Autodesk Fusion 360 part; units mm, degrees
(part 2 of 2)
  spline S93 degree 3 poles (-0.4829, 17.1605) (-0.5355, 17.2267) (-0.6438, 17.3632) (-0.6565, 17.5373) (-0.663, 17.6271) knots 0 0 0 0 0.024747 0.051056 0.051056 0.051056 0.051056
  spline S94 degree 3 poles (-0.663, 17.6271) (-0.6569, 17.7139) (-0.645, 17.8842) (-0.5509, 18.0265) (-0.5048, 18.0964) knots 0 0 0 0 0.025614 0.050281 0.050281 0.050281 0.050281
  spline S95 degree 3 poles (-0.5048, 18.0964) (-0.4337, 18.1672) (-0.2885, 18.3119) (-0.0839, 18.33) (0.0205, 18.3392) knots 0 0 0 0 0.029141 0.059529 0.059529 0.059529 0.059529
  line L42 (4.4066, 19.7731) -> (4.2483, 19.7731)
  line L43 (4.2483, 19.7731) -> (4.2483, 21.7813)
  line L44 (4.2483, 21.7813) -> (4.4939, 21.7813)
  line L45 (4.4939, 21.7813) -> (4.4939, 20.2164)
  spline S96 degree 3 poles (4.4939, 20.2164) (4.5274, 20.2456) (4.5999, 20.3087) (4.6822, 20.3587) (4.7265, 20.3856) knots 0 0 0 0 0.013289 0.028808 0.028808 0.028808 0.028808
  spline S97 degree 3 poles (4.7265, 20.3856) (4.7715, 20.4114) (4.855, 20.4592) (4.944, 20.4957) (4.985, 20.5125) knots 0 0 0 0 0.015536 0.028826 0.028826 0.028826 0.028826
  line L46 (4.985, 20.5125) -> (4.985, 20.2751)
  spline S98 degree 3 poles (4.985, 20.2751) (4.9192, 20.2417) (4.7906, 20.1765) (4.6792, 20.0851) (4.6249, 20.0405) knots 0 0 0 0 0.022076 0.0431 0.0431 0.0431 0.0431
  spline S99 degree 3 poles (4.6249, 20.0405) (4.5785, 19.9972) (4.4934, 19.918) (4.4337, 19.8184) (4.4066, 19.7731) knots 0 0 0 0 0.01891 0.03467 0.03467 0.03467 0.03467
  spline S100 degree 3 poles (-4.5976, 21.8167) (-4.5145, 21.8111) (-4.3537, 21.8001) (-4.2234, 21.7056) (-4.1603, 21.6598) knots 0 0 0 0 0.024413 0.047298 0.047298 0.047298 0.047298
  spline S101 degree 3 poles (-4.1603, 21.6598) (-4.1085, 21.6029) (-4.0028, 21.4869) (-3.9757, 21.3321) (-3.9618, 21.2533) knots 0 0 0 0 0.022603 0.04608 0.04608 0.04608 0.04608
  line L47 (-3.9618, 21.2533) -> (-4.2074, 21.2205)
  spline S102 degree 3 poles (-4.2074, 21.2205) (-4.2215, 21.2828) (-4.2469, 21.3945) (-4.3193, 21.4825) (-4.3513, 21.5214) knots 0 0 0 0 0.018844 0.033755 0.033755 0.033755 0.033755
  spline S103 degree 3 poles (-4.3513, 21.5214) (-4.3875, 21.5482) (-4.461, 21.6029) (-4.5524, 21.6099) (-4.5989, 21.6134) knots 0 0 0 0 0.01322 0.026904 0.026904 0.026904 0.026904
  spline S104 degree 3 poles (-4.5989, 21.6134) (-4.6543, 21.6086) (-4.7643, 21.5989) (-4.8493, 21.5284) (-4.8916, 21.4934) knots 0 0 0 0 0.016258 0.032307 0.032307 0.032307 0.032307
  spline S105 degree 3 poles (-4.8916, 21.4934) (-4.9264, 21.4506) (-4.9969, 21.3639) (-5.0062, 21.2524) (-5.0109, 21.196) knots 0 0 0 0 0.016147 0.032721 0.032721 0.032721 0.032721
  spline S106 degree 3 poles (-5.0109, 21.196) (-5.0068, 21.1425) (-4.9986, 21.038) (-4.9327, 20.9567) (-4.9004, 20.917) knots 0 0 0 0 0.015678 0.030648 0.030648 0.030648 0.030648
  spline S107 degree 3 poles (-4.9004, 20.917) (-4.8604, 20.885) (-4.7783, 20.8193) (-4.6732, 20.8113) (-4.6194, 20.8072) knots 0 0 0 0 0.015012 0.030805 0.030805 0.030805 0.030805
  spline S108 degree 3 poles (-4.6194, 20.8072) (-4.5933, 20.8087) (-4.5347, 20.8122) (-4.4777, 20.8265) (-4.4461, 20.8345) knots 0 0 0 0 0.00784 0.017573 0.017573 0.017573 0.017573
  line L48 (-4.4461, 20.8345) -> (-4.4734, 20.6189)
  spline S109 degree 3 poles (-4.4734, 20.6189) (-4.4808, 20.6197) (-4.494, 20.6211) (-4.5072, 20.6215) (-4.513, 20.6216) knots 0 0 0 0 0.002226 0.003967 0.003967 0.003967 0.003967
  spline S110 degree 3 poles (-4.513, 20.6216) (-4.5637, 20.6184) (-4.6639, 20.612) (-4.7519, 20.5637) (-4.7954, 20.5398) knots 0 0 0 0 0.015044 0.029725 0.029725 0.029725 0.029725
  spline S111 degree 3 poles (-4.7954, 20.5398) (-4.832, 20.5078) (-4.9081, 20.4411) (-4.9165, 20.34) (-4.9209, 20.2874) knots 0 0 0 0 0.014029 0.029194 0.029194 0.029194 0.029194
  spline S112 degree 3 poles (-4.9209, 20.2874) (-4.9173, 20.2446) (-4.9104, 20.1603) (-4.8561, 20.0955) (-4.8295, 20.0637) knots 0 0 0 0 0.012556 0.024703 0.024703 0.024703 0.024703
  spline S113 degree 3 poles (-4.8295, 20.0637) (-4.796, 20.0378) (-4.7266, 19.9842) (-4.6389, 19.9781) (-4.5935, 19.975) knots 0 0 0 0 0.012404 0.025721 0.025721 0.025721 0.025721
  spline S114 degree 3 poles (-4.5935, 19.975) (-4.5481, 19.9783) (-4.4596, 19.9849) (-4.3891, 20.0388) (-4.3547, 20.065) knots 0 0 0 0 0.013323 0.026012 0.026012 0.026012 0.026012
  spline S115 degree 3 poles (-4.3547, 20.065) (-4.3254, 20.1011) (-4.2612, 20.1801) (-4.2423, 20.2805) (-4.2319, 20.3351) knots 0 0 0 0 0.013719 0.030088 0.030088 0.030088 0.030088
  line L49 (-4.2319, 20.3351) -> (-3.9864, 20.2915)
  spline S116 degree 3 poles (-3.9864, 20.2915) (-4.0047, 20.2151) (-4.0397, 20.0694) (-4.1423, 19.9605) (-4.191, 19.9088) knots 0 0 0 0 0.023119 0.04407 0.04407 0.04407 0.04407
  spline S117 degree 3 poles (-4.191, 19.9088) (-4.2487, 19.8692) (-4.3683, 19.7873) (-4.5131, 19.7779) (-4.588, 19.7731) knots 0 0 0 0 0.020598 0.042654 0.042654 0.042654 0.042654
  spline S118 degree 3 poles (-4.588, 19.7731) (-4.6412, 19.7758) (-4.7459, 19.7812) (-4.8421, 19.8228) (-4.8895, 19.8433) knots 0 0 0 0 0.015821 0.03118 0.03118 0.03118 0.03118
  spline S119 degree 3 poles (-4.8895, 19.8433) (-4.9324, 19.8684) (-5.0164, 19.9174) (-5.0728, 19.9964) (-5.1003, 20.035) knots 0 0 0 0 0.014725 0.02878 0.02878 0.02878 0.02878
  spline S120 degree 3 poles (-5.1003, 20.035) (-5.1216, 20.0759) (-5.1637, 20.1568) (-5.1701, 20.2478) (-5.1733, 20.2928) knots 0 0 0 0 0.013662 0.027054 0.027054 0.027054 0.027054
  spline S121 degree 3 poles (-5.1733, 20.2928) (-5.1704, 20.335) (-5.1648, 20.4188) (-5.124, 20.4923) (-5.1037, 20.5289) knots 0 0 0 0 0.012502 0.024877 0.024877 0.024877 0.024877
  spline S122 degree 3 poles (-5.1037, 20.5289) (-5.0768, 20.5629) (-5.0205, 20.6342) (-4.9398, 20.6761) (-4.8977, 20.698) knots 0 0 0 0 0.012871 0.026927 0.026927 0.026927 0.026927
  spline S123 degree 3 poles (-4.8977, 20.698) (-4.953, 20.7146) (-5.0601, 20.7468) (-5.1364, 20.8284) (-5.1733, 20.8679) knots 0 0 0 0 0.016967 0.032892 0.032892 0.032892 0.032892
  spline S124 degree 3 poles (-5.1733, 20.8679) (-5.2019, 20.915) (-5.2621, 21.0139) (-5.2683, 21.1298) (-5.2715, 21.1905) knots 0 0 0 0 0.016275 0.034197 0.034197 0.034197 0.034197
  spline S125 degree 3 poles (-5.2715, 21.1905) (-5.2635, 21.2746) (-5.2474, 21.443) (-5.1362, 21.5707) (-5.0805, 21.6346) knots 0 0 0 0 0.024665 0.049435 0.049435 0.049435 0.049435
  spline S126 degree 3 poles (-5.0805, 21.6346) (-5.0113, 21.6877) (-4.869, 21.797) (-4.6897, 21.81) (-4.5976, 21.8167) knots 0 0 0 0 0.025577 0.052634 0.052634 0.052634 0.052634
  spline S127 degree 3 poles (0, 25.2779) (0.0905, 25.2701) (0.267, 25.2551) (0.3929, 25.131) (0.4543, 25.0705) knots 0 0 0 0 0.026334 0.051363 0.051363 0.051363 0.051363
  spline S128 degree 3 poles (0.4543, 25.0705) (0.5117, 24.9633) (0.6467, 24.7108) (0.6501, 24.423) (0.6521, 24.2574) knots 0 0 0 0 0.036009 0.08476 0.08476 0.08476 0.08476
  spline S129 degree 3 poles (0.6521, 24.2574) (0.6507, 24.1501) (0.6481, 23.9568) (0.6003, 23.7697) (0.5791, 23.6865) knots 0 0 0 0 0.032061 0.057736 0.057736 0.057736 0.057736
  spline S130 degree 3 poles (0.5791, 23.6865) (0.5533, 23.6197) (0.5043, 23.4931) (0.4078, 23.3979) (0.3622, 23.3529) knots 0 0 0 0 0.021191 0.040192 0.040192 0.040192 0.040192
  spline S131 degree 3 poles (0.3622, 23.3529) (0.3097, 23.3187) (0.1997, 23.2471) (0.0685, 23.2395) (0, 23.2356) knots 0 0 0 0 0.018481 0.038665 0.038665 0.038665 0.038665
  spline S132 degree 3 poles (0, 23.2356) (-0.0511, 23.2378) (-0.1493, 23.2421) (-0.2393, 23.2815) (-0.2824, 23.3004) knots 0 0 0 0 0.015196 0.029197 0.029197 0.029197 0.029197
  spline S133 degree 3 poles (-0.2824, 23.3004) (-0.3213, 23.3246) (-0.4002, 23.3739) (-0.4551, 23.4491) (-0.4829, 23.4873) knots 0 0 0 0 0.013619 0.027641 0.027641 0.027641 0.027641
  spline S134 degree 3 poles (-0.4829, 23.4873) (-0.5083, 23.5316) (-0.5619, 23.6256) (-0.5915, 23.7297) (-0.6071, 23.7847) knots 0 0 0 0 0.01527 0.032333 0.032333 0.032333 0.032333
  spline S135 degree 3 poles (-0.6071, 23.7847) (-0.6202, 23.8531) (-0.65, 24.0091) (-0.6514, 24.1681) (-0.6521, 24.2574) knots 0 0 0 0 0.020858 0.04757 0.04757 0.04757 0.04757
  spline S136 degree 3 poles (-0.6521, 24.2574) (-0.6507, 24.364) (-0.648, 24.5564) (-0.6008, 24.7426) (-0.5798, 24.8256) knots 0 0 0 0 0.031856 0.057454 0.057454 0.057454 0.057454
  spline S137 degree 3 poles (-0.5798, 24.8256) (-0.5541, 24.8924) (-0.5054, 25.0192) (-0.4091, 25.1147) (-0.3636, 25.1598) knots 0 0 0 0 0.021185 0.040213 0.040213 0.040213 0.040213
  spline S138 degree 3 poles (-0.3636, 25.1598) (-0.3109, 25.1942) (-0.2006, 25.2663) (-0.0689, 25.2739) (0, 25.2779) knots 0 0 0 0 0.018535 0.038823 0.038823 0.038823 0.038823
  arc A0 (6.725, 12.125) -> (6.925, 12.325) centre (6.725, 12.325) ccw
  line L50 (6.925, 12.325) -> (6.925, 25.775)
  arc A1 (6.925, 25.775) -> (6.725, 25.975) centre (6.725, 25.775) ccw
  line L51 (6.725, 25.975) -> (-6.725, 25.975)
  arc A2 (-6.725, 25.975) -> (-6.925, 25.775) centre (-6.725, 25.775) ccw
  line L52 (-6.925, 25.775) -> (-6.925, 12.325)
  arc A3 (-6.925, 12.325) -> (-6.725, 12.125) centre (-6.725, 12.325) ccw
  line L53 (-6.725, 12.125) -> (6.725, 12.125)
  spline S139 degree 3 poles (0.0027, 23.4388) (0.0564, 23.4451) (0.165, 23.4576) (0.2367, 23.5403) (0.2729, 23.5821) knots 0 0 0 0 0.015627 0.031586 0.031586 0.031586 0.031586
  spline S140 degree 3 poles (0.2729, 23.5821) (0.3095, 23.6678) (0.4012, 23.8822) (0.4003, 24.1166) (0.3997, 24.2574) knots 0 0 0 0 0.027708 0.069337 0.069337 0.069337 0.069337
  spline S141 degree 3 poles (0.3997, 24.2574) (0.4011, 24.3964) (0.4034, 24.6233) (0.3177, 24.832) (0.2844, 24.9129) knots 0 0 0 0 0.041114 0.067132 0.067132 0.067132 0.067132
  spline S142 degree 3 poles (0.2844, 24.9129) (0.2453, 24.9604) (0.1706, 25.051) (0.055, 25.0679) (0, 25.0759) knots 0 0 0 0 0.017756 0.03385 0.03385 0.03385 0.03385
  spline S143 degree 3 poles (0, 25.0759) (-0.055, 25.0679) (-0.1708, 25.0508) (-0.2453, 24.9599) (-0.2844, 24.9122) knots 0 0 0 0 0.016099 0.03389 0.03389 0.03389 0.03389
  spline S144 degree 3 poles (-0.2844, 24.9122) (-0.3177, 24.8313) (-0.4033, 24.6228) (-0.4011, 24.3961) (-0.3997, 24.2574) knots 0 0 0 0 0.026034 0.067063 0.067063 0.067063 0.067063
  spline S145 degree 3 poles (-0.3997, 24.2574) (-0.4012, 24.1181) (-0.4035, 23.8909) (-0.3177, 23.682) (-0.2844, 23.6012) knots 0 0 0 0 0.041199 0.067201 0.067201 0.067201 0.067201
  spline S146 degree 3 poles (-0.2844, 23.6012) (-0.245, 23.5539) (-0.1694, 23.4632) (-0.053, 23.4467) (0.0027, 23.4388) knots 0 0 0 0 0.01777 0.034058 0.034058 0.034058 0.034058
  line L54 (4.4407, 16.713) -> (5.0669, 17.6148)
  line L55 (5.0669, 17.6148) -> (4.4407, 17.6148)
  line L56 (4.4407, 17.6148) -> (4.4407, 16.713)
  spline S147 degree 3 poles (-4.6371, 17.2383) (-4.5838, 17.2432) (-4.477, 17.2532) (-4.3955, 17.3228) (-4.3547, 17.3576) knots 0 0 0 0 0.015669 0.031337 0.031337 0.031337 0.031337
  spline S148 degree 3 poles (-4.3547, 17.3576) (-4.3209, 17.4018) (-4.2503, 17.494) (-4.2427, 17.6102) (-4.2388, 17.6707) knots 0 0 0 0 0.016309 0.034061 0.034061 0.034061 0.034061
  spline S149 degree 3 poles (-4.2388, 17.6707) (-4.241, 17.7126) (-4.2456, 17.7965) (-4.2769, 17.8745) (-4.2927, 17.9136) knots 0 0 0 0 0.012488 0.025026 0.025026 0.025026 0.025026
  spline S150 degree 3 poles (-4.2927, 17.9136) (-4.3119, 17.9496) (-4.3493, 18.0196) (-4.4127, 18.0672) (-4.4434, 18.0902) knots 0 0 0 0 0.012088 0.023476 0.023476 0.023476 0.023476
  spline S151 degree 3 poles (-4.4434, 18.0902) (-4.4757, 18.1079) (-4.5392, 18.1427) (-4.6113, 18.1482) (-4.6467, 18.1509) knots 0 0 0 0 0.01092 0.021432 0.021432 0.021432 0.021432
  spline S152 degree 3 poles (-4.6467, 18.1509) (-4.6971, 18.1453) (-4.8002, 18.1336) (-4.8756, 18.062) (-4.9141, 18.0254) knots 0 0 0 0 0.014798 0.030269 0.030269 0.030269 0.030269
  spline S153 degree 3 poles (-4.9141, 18.0254) (-4.9467, 17.9777) (-5.0166, 17.8752) (-5.0227, 17.7508) (-5.0259, 17.6844) knots 0 0 0 0 0.017015 0.03652 0.03652 0.03652 0.03652
  spline S154 degree 3 poles (-5.0259, 17.6844) (-5.0227, 17.6205) (-5.0166, 17.5007) (-4.9476, 17.4031) (-4.9154, 17.3576) knots 0 0 0 0 0.018742 0.035129 0.035129 0.035129 0.035129
  spline S155 degree 3 poles (-4.9154, 17.3576) (-4.876, 17.3228) (-4.7963, 17.2526) (-4.6905, 17.2431) (-4.6371, 17.2383) knots 0 0 0 0 0.015362 0.030997 0.030997 0.030997 0.030997
  spline S156 degree 3 poles (-4.6112, 13.9613) (-4.6653, 13.9566) (-4.7718, 13.9474) (-4.852, 13.8767) (-4.8916, 13.8419) knots 0 0 0 0 0.01582 0.031195 0.031195 0.031195 0.031195
  spline S157 degree 3 poles (-4.8916, 13.8419) (-4.9236, 13.796) (-4.9926, 13.697) (-4.9983, 13.576) (-5.0014, 13.5111) knots 0 0 0 0 0.01645 0.035493 0.035493 0.035493 0.035493
  spline S158 degree 3 poles (-5.0014, 13.5111) (-4.998, 13.4458) (-4.9917, 13.323) (-4.9216, 13.2225) (-4.8888, 13.1755) knots 0 0 0 0 0.019171 0.036033 0.036033 0.036033 0.036033
  spline S159 degree 3 poles (-4.8888, 13.1755) (-4.8499, 13.1393) (-4.7732, 13.068) (-4.6692, 13.0568) (-4.618, 13.0513) knots 0 0 0 0 0.015505 0.030512 0.030512 0.030512 0.030512
  spline S160 degree 3 poles (-4.618, 13.0513) (-4.5647, 13.0575) (-4.4549, 13.0702) (-4.3743, 13.1461) (-4.3329, 13.185) knots 0 0 0 0 0.015674 0.03225 0.03225 0.03225 0.03225
  spline S161 degree 3 poles (-4.3329, 13.185) (-4.2975, 13.2344) (-4.2234, 13.3378) (-4.2156, 13.465) (-4.2115, 13.5316) knots 0 0 0 0 0.017846 0.037388 0.037388 0.037388 0.037388
  spline S162 degree 3 poles (-4.2115, 13.5316) (-4.2155, 13.5914) (-4.2232, 13.7065) (-4.2932, 13.798) (-4.3268, 13.8419) knots 0 0 0 0 0.017547 0.033771 0.033771 0.033771 0.033771
  spline S163 degree 3 poles (-4.3268, 13.8419) (-4.3676, 13.8767) (-4.4497, 13.9468) (-4.5572, 13.9564) (-4.6112, 13.9613) knots 0 0 0 0 0.015682 0.031535 0.031535 0.031535 0.031535
  spline S164 degree 3 poles (0.0055, 13.8781) (0.0603, 13.8825) (0.168, 13.8911) (0.2516, 13.9593) (0.2926, 13.9927) knots 0 0 0 0 0.016099 0.03158 0.03158 0.03158 0.03158
  spline S165 degree 3 poles (0.2926, 13.9927) (0.3259, 14.0337) (0.3935, 14.1173) (0.4021, 14.2246) (0.4065, 14.2792) knots 0 0 0 0 0.015466 0.031479 0.031479 0.031479 0.031479
  spline S166 degree 3 poles (0.4065, 14.2792) (0.4044, 14.3141) (0.4, 14.3848) (0.3713, 14.4496) (0.3568, 14.4824) knots 0 0 0 0 0.010409 0.021077 0.021077 0.021077 0.021077
  spline S167 degree 3 poles (0.3568, 14.4824) (0.3381, 14.5134) (0.3005, 14.5755) (0.2394, 14.6148) (0.2087, 14.6346) knots 0 0 0 0 0.010689 0.021477 0.021477 0.021477 0.021477
  spline S168 degree 3 poles (0.2087, 14.6346) (0.1753, 14.6503) (0.1083, 14.6818) (0.0343, 14.6862) (-0.0027, 14.6884) knots 0 0 0 0 0.01097 0.022 0.022 0.022 0.022
  spline S169 degree 3 poles (-0.0027, 14.6884) (-0.0583, 14.6842) (-0.1669, 14.676) (-0.2519, 14.6082) (-0.2933, 14.5752) knots 0 0 0 0 0.016312 0.031835 0.031835 0.031835 0.031835
  spline S170 degree 3 poles (-0.2933, 14.5752) (-0.3267, 14.5343) (-0.3951, 14.4505) (-0.4036, 14.3426) (-0.4079, 14.2874) knots 0 0 0 0 0.015466 0.031649 0.031649 0.031649 0.031649
  spline S171 degree 3 poles (-0.4079, 14.2874) (-0.4034, 14.2312) (-0.3945, 14.121) (-0.3243, 14.0358) (-0.2899, 13.994) knots 0 0 0 0 0.016467 0.032302 0.032302 0.032302 0.032302
  spline S172 degree 3 poles (-0.2899, 13.994) (-0.2475, 13.9602) (-0.1611, 13.8912) (-0.0508, 13.8825) (0.0055, 13.8781) knots 0 0 0 0 0.015878 0.032386 0.032386 0.032386 0.032386
  spline S173 degree 3 poles (0.0014, 13.05) (0.0458, 13.0534) (0.1328, 13.06) (0.2012, 13.1138) (0.2347, 13.14) knots 0 0 0 0 0.013054 0.025513 0.025513 0.025513 0.025513
  spline S174 degree 3 poles (0.2347, 13.14) (0.2617, 13.1713) (0.3154, 13.2334) (0.3234, 13.3151) (0.3274, 13.3556) knots 0 0 0 0 0.012093 0.023986 0.023986 0.023986 0.023986
  spline S175 degree 3 poles (0.3274, 13.3556) (0.3241, 13.4002) (0.3175, 13.4872) (0.2627, 13.5547) (0.236, 13.5875) knots 0 0 0 0 0.013093 0.025466 0.025466 0.025466 0.025466
  spline S176 degree 3 poles (0.236, 13.5875) (0.2025, 13.6137) (0.1328, 13.6682) (0.0444, 13.6744) (-0.0014, 13.6775) knots 0 0 0 0 0.012488 0.025912 0.025912 0.025912 0.025912
  spline S177 degree 3 poles (-0.0014, 13.6775) (-0.046, 13.6743) (-0.1328, 13.668) (-0.2009, 13.6142) (-0.234, 13.5882) knots 0 0 0 0 0.013101 0.025433 0.025433 0.025433 0.025433
  spline S178 degree 3 poles (-0.234, 13.5882) (-0.2604, 13.5566) (-0.3136, 13.4932) (-0.321, 13.4107) (-0.3247, 13.3692) knots 0 0 0 0 0.012047 0.024215 0.024215 0.024215 0.024215
  spline S179 degree 3 poles (-0.3247, 13.3692) (-0.3209, 13.3261) (-0.3135, 13.2406) (-0.2585, 13.1747) (-0.2312, 13.1421) knots 0 0 0 0 0.012649 0.025094 0.025094 0.025094 0.025094
  spline S180 degree 3 poles (-0.2312, 13.1421) (-0.1978, 13.1152) (-0.1298, 13.0606) (-0.0428, 13.0536) (0.0014, 13.05) knots 0 0 0 0 0.012558 0.025536 0.025536 0.025536 0.025536
sketch "Sketch1 (3)" plane through (0, 0, -5) normal (0, 0, -1) x (1, 0, 0) in component "Case"
  arc A0 (63.55, -96.125) -> (66.55, -93.125) centre (63.55, -93.125) ccw
  line L0 (66.55, -93.125) -> (66.55, 33.075)
  arc A1 (66.55, 33.075) -> (63.55, 36.075) centre (63.55, 33.075) ccw
  line L1 (63.55, 36.075) -> (-25.45, 36.075)
  arc A2 (-25.45, 36.075) -> (-28.45, 33.075) centre (-25.45, 33.075) ccw
  line L2 (-28.45, 33.075) -> (-28.45, -93.125)
  arc A3 (-28.45, -93.125) -> (-25.45, -96.125) centre (-25.45, -93.125) ccw
  line L3 (-25.45, -96.125) -> (63.55, -96.125)
  circle A4 centre (-18.45, -83.625) radius 2
  circle A5 centre (-18.45, -52.625) radius 2
  circle A6 centre (56.55, -52.625) radius 2
  circle A7 centre (-23.45, 31.075) radius 2
  circle A8 centre (-23.45, -91.125) radius 2
  circle A9 centre (61.55, 31.075) radius 2
  circle A10 centre (56.55, -83.625) radius 2
  line L4 (-10.025, 9.025) -> (10.025, 9.025)
  line L5 (10.025, 9.025) -> (10.025, 29.075)
  line L6 (10.025, 29.075) -> (48.125, 29.075)
  line L7 (48.125, 29.075) -> (48.125, -48.125)
  line L8 (48.125, -48.125) -> (-10.025, -48.125)
  line L9 (-10.025, -48.125) -> (-10.025, 9.025)
  line L10 (-16.95, -55.625) -> (55.05, -55.625)
  line L11 (55.05, -55.625) -> (55.05, -80.625)
  line L12 (55.05, -80.625) -> (-16.95, -80.625)
  line L13 (-16.95, -80.625) -> (-16.95, -55.625)
  circle A11 centre (61.55, -91.125) radius 2
  line L14 (61.55, -91.125) -> (61.55, 31.075)
  line L15 (61.55, 31.075) -> (-23.45, 31.075)
  line L16 (-23.45, 31.075) -> (-23.45, -91.125)
  line L17 (-23.45, -91.125) -> (61.55, -91.125)
  circle A12 centre (61.55, -91.125) radius 2.3
  circle A13 centre (-23.45, -91.125) radius 2.3
  circle A14 centre (-23.45, 31.075) radius 2.3
  circle A15 centre (61.55, 31.075) radius 2.3
  circle A16 centre (61.55, -91.125) radius 5.0139
  circle A17 centre (56.55, -83.625) radius 4
  circle A18 centre (-23.45, -91.125) radius 5.0139
  circle A19 centre (-23.45, 31.075) radius 5.0139
  circle A20 centre (61.55, 31.075) radius 5.0139
  dimension "d103" = 4.6
  dimension "d104" = 8
  constraint concentric A11 A12
  constraint concentric A8 A13
  constraint concentric A7 A14
  constraint concentric A9 A15
  constraint equal A14 A15
  constraint equal A13 A14
  constraint equal A12 A13
  constraint concentric A11 A16
  constraint concentric A10 A17
  constraint tangent A16 A17
  constraint concentric A13 A18
  constraint concentric A14 A19
  constraint concentric A15 A20
  constraint equal A19 A20
  constraint equal A18 A19
  constraint equal A16 A18
  measures "d103" diameter of A12
  measures "d104" diameter of A17
extrude "Extrude1''" add sketch "Sketch1 (3)" along normal blind 6 separate body contours A0 L0 L3 A16 | L0 L3 L14 L17 A12 A16 | L3 L17 A16 A18 | L0 L14 A16 A20 | L2 L3 L16 L17 A13 A18 | L14 L17 A12 A16 | L0 L1 L14 L15 A15 A20 | L2 A3 L3 A18 | L16 L17 A13 A18 | L0 A1 L1 A20 | L14 L15 A15 A20 | L2 L16 A18 A19 | L1 L15 A19 A20 | L1 L2 L15 L16 A14 A19 | L15 L16 A14 A19 | L1 A2 L2 A19 makes body 3 in component "Case"
sketch "Sketch2 (2)" plane through (0, 0, -11) normal (0, 0, -1) x (1, 0, 0) in component "Case"
  circle A0 centre (-23.45, 31.075) radius 2.3
  circle A1 centre (61.55, -91.125) radius 2.3
  circle A2 centre (61.55, 31.075) radius 2.3
  circle A3 centre (-23.45, -91.125) radius 2.3
  line L0 (56.5361, -91.125) -> (-18.4361, -91.125)
  arc A4 (-18.4361, -91.125) -> (-23.45, -86.1111) centre (-23.45, -91.125) ccw
  line L1 (-23.45, -86.1111) -> (-23.45, 26.0611)
  arc A5 (-23.45, 26.0611) -> (-18.4361, 31.075) centre (-23.45, 31.075) ccw
  line L2 (-18.4361, 31.075) -> (56.5361, 31.075)
  arc A6 (56.5361, 31.075) -> (61.55, 26.0611) centre (61.55, 31.075) ccw
  line L3 (61.55, 26.0611) -> (61.55, -86.1111)
  arc A7 (61.55, -86.1111) -> (56.5361, -91.125) centre (61.55, -91.125) ccw
  line L4 (-25.45, -96.125) -> (63.55, -96.125)
  arc A8 (63.55, -96.125) -> (66.55, -93.125) centre (63.55, -93.125) ccw
  line L5 (66.55, -93.125) -> (66.55, 33.075)
  arc A9 (66.55, 33.075) -> (63.55, 36.075) centre (63.55, 33.075) ccw
  line L6 (63.55, 36.075) -> (-25.45, 36.075)
  arc A10 (-25.45, 36.075) -> (-28.45, 33.075) centre (-25.45, 33.075) ccw
  line L7 (-28.45, 33.075) -> (-28.45, -93.125)
  arc A11 (-28.45, -93.125) -> (-25.45, -96.125) centre (-25.45, -93.125) ccw
extrude "Extrude2''" add sketch "Sketch2 (2)" along normal blind 60 contours A0 | A1 | A2 | A3 | L4 A8 L5 A9 L6 A10 L7 A11 bodies 3 in component "Case"
sketch "Sketch3" plane through (0, 0, -71) normal (0, 0, -1) x (1, 0, 0) in component "Case"
  line L0 (61.55, 26.0611) -> (61.55, -86.1111)
  arc A0 (61.55, -86.1111) -> (56.5361, -91.125) centre (61.55, -91.125) ccw
  line L1 (56.5361, -91.125) -> (-18.4361, -91.125)
  arc A1 (-18.4361, -91.125) -> (-23.45, -86.1111) centre (-23.45, -91.125) ccw
  line L2 (-23.45, -86.1111) -> (-23.45, 26.0611)
  arc A2 (-23.45, 26.0611) -> (-18.4361, 31.075) centre (-23.45, 31.075) ccw
  line L3 (-18.4361, 31.075) -> (56.5361, 31.075)
  arc A3 (56.5361, 31.075) -> (61.55, 26.0611) centre (61.55, 31.075) ccw
  arc A4 (-28.45, -93.125) -> (-25.45, -96.125) centre (-25.45, -93.125) ccw
  line L4 (-25.45, -96.125) -> (63.55, -96.125)
  arc A5 (63.55, -96.125) -> (66.55, -93.125) centre (63.55, -93.125) ccw
  line L5 (66.55, -93.125) -> (66.55, 33.075)
  arc A6 (66.55, 33.075) -> (63.55, 36.075) centre (63.55, 33.075) ccw
  line L6 (63.55, 36.075) -> (-25.45, 36.075)
  arc A7 (-25.45, 36.075) -> (-28.45, 33.075) centre (-25.45, 33.075) ccw
  line L7 (-28.45, 33.075) -> (-28.45, -93.125)
extrude "Extrude3" add sketch "Sketch3" along normal blind 5 contours L0 A0 L1 A1 L2 A2 L3 A3 | A4 L4 A5 L5 A6 L6 A7 L7 bodies 3 in component "Case"
sketch "Sketch4 (2)" plane through (0, 0, -71) normal (0, 0, 1) x (-1, 0, 0) in component "Case"
  arc A0 (-56.5361, -91.125) -> (-61.55, -86.1111) centre (-61.55, -91.125) ccw
  line L0 (-56.5361, -91.125) -> (18.4361, -91.125)
  arc A1 (23.45, -86.1111) -> (18.4361, -91.125) centre (23.45, -91.125) ccw
  line L1 (23.45, -86.1111) -> (23.45, 26.0611)
  arc A2 (18.4361, 31.075) -> (23.45, 26.0611) centre (23.45, 31.075) ccw
  line L2 (18.4361, 31.075) -> (-56.5361, 31.075)
  arc A3 (-61.55, 26.0611) -> (-56.5361, 31.075) centre (-61.55, 31.075) ccw
  line L3 (-61.55, 26.0611) -> (-61.55, -86.1111)
  line L4 (8.65, -53.1111) -> (-61.35, -53.1111)
  line L5 (-61.35, -53.1111) -> (-61.35, -83.1111)
  line L6 (-61.35, -83.1111) -> (8.65, -83.1111)
  line L7 (8.65, -83.1111) -> (8.65, -53.1111)
  line L8 (8.65, -53.1111) -> (-61.35, -83.1111) construction
  line L9 (-61.35, -53.1111) -> (8.65, -83.1111) construction
  line L10 (-61.35, -74.1111) -> (-53.35, -74.1111)
  line L11 (-53.35, -74.1111) -> (-53.35, -65.1111)
  line L12 (-53.35, -65.1111) -> (-61.35, -65.1111)
  line L13 (-61.35, -83.1111) -> (-61.55, -83.1111) construction
  line L14 (-61.55, -83.1111) -> (-61.55, -86.1111) construction
  line L15 (-61.55, -86.1111) -> (-61.35, -86.1111) construction
  line L16 (-61.35, -86.1111) -> (-61.35, -83.1111) construction
  line L17 (6.555, -81.1061) -> (-59.255, -81.1061) construction
  line L18 (-59.255, -81.1061) -> (-59.255, -55.1161) construction
  line L19 (-59.255, -55.1161) -> (6.555, -55.1161) construction
  line L20 (6.555, -55.1161) -> (6.555, -81.1061) construction
  line L21 (6.555, -81.1061) -> (-59.255, -55.1161) construction
  line L22 (-59.255, -81.1061) -> (6.555, -55.1161) construction
  circle A4 centre (6.555, -81.1061) radius 1.15
  circle A5 centre (-59.255, -81.1061) radius 1.15
  circle A6 centre (-59.255, -55.1161) radius 1.15
  circle A7 centre (6.555, -55.1161) radius 1.15
  circle A8 centre (6.555, -81.1061) radius 3.65
  circle A9 centre (-59.255, -81.1061) radius 3.65
  circle A10 centre (-59.255, -55.1161) radius 3.65
  circle A11 centre (6.555, -55.1161) radius 3.65
  circle A12 centre (13.855, -6.055) radius 3.65
  line L23 (13.855, -6.055) -> (13.855, -32.045) construction
  circle A13 centre (-51.955, -32.045) radius 1.15
  circle A14 centre (-51.955, -6.055) radius 1.15
  line L24 (13.855, -32.045) -> (-51.955, -6.055) construction
  line L25 (-54.05, -4.05) -> (15.95, -34.05) construction
  line L26 (-51.955, -32.045) -> (-51.955, -6.055) construction
  circle A15 centre (-51.955, -32.045) radius 3.65
  circle A16 centre (13.855, -32.045) radius 1.15
  line L27 (15.95, -4.05) -> (-54.05, -34.05) construction
  line L28 (13.855, -32.045) -> (-51.955, -32.045) construction
  circle A17 centre (-51.955, -6.055) radius 3.65
  line L29 (-51.955, -6.055) -> (13.855, -6.055) construction
  line L30 (15.95, -4.05) -> (-54.05, -4.05)
  circle A18 centre (13.855, -32.045) radius 3.65
  line L31 (-54.05, -4.05) -> (-54.05, -34.05)
  circle A19 centre (13.855, -6.055) radius 1.15
  line L32 (15.95, -34.05) -> (15.95, -4.05)
  line L33 (-54.05, -34.05) -> (15.95, -34.05)
  line L34 (-51.955, -32.045) -> (13.855, -6.055) construction
  line L35 (-26.075, -25.775) -> (-26.075, -12.325) construction
  line L36 (-12.025, -12.325) -> (-12.025, -25.775) construction
  line L37 (-26.075, -12.325) -> (-12.025, -25.775) construction
  line L38 (-12.025, -12.325) -> (-26.075, -25.775) construction
  point P0 (-26.35, -68.1111)
  point P1 (-26.35, -68.1111)
  point P2 (-19.05, -19.05)
  point P3 (-19.05, -19.05)
  point P4 (-19.05, -19.05)
  dimension "d111" = 70
  dimension "d112" = 30
  dimension "d113" = 9
  dimension "d114" = 9
  dimension "d115" = 8
  dimension "d116" = 3
  dimension "d117" = 0.2
  dimension "d118" = 65.81
  dimension "d119" = 25.99
  dimension "d122" = 2.3
  dimension "d123" = 2.5
  dimension "d135" = 2.5
  dimension "d136" = 70
  dimension "d137" = 30
  dimension "d143" = 65.81
  dimension "d144" = 25.99
  dimension "d145" = 2.3
  constraint horizontal L4
  constraint perpendicular L4 L5
  constraint parallel L4 L6
  constraint parallel L5 L7
  constraint coincident L8 P1
  constraint coincident L9 P1
  constraint coincident L5 L10.start
  constraint perpendicular L5 L10
  constraint perpendicular L10 L11
  constraint perpendicular L5 L12
  constraint coincident L5 L12.end
  constraint horizontal L13
  constraint vertical L14
  constraint horizontal L15
  constraint vertical L16
  constraint coincident A0.end L3.end
  constraint horizontal L17
  constraint perpendicular L17 L18
  constraint parallel L17 L19
  constraint parallel L18 L20
  constraint coincident L21 P1
  constraint coincident L22 P1
  constraint coincident L17.start L20.end
  constraint coincident L17.end L18.start
  constraint coincident L18.end L19.start
  constraint coincident L19.end L20.start
  constraint equal A6 A7
  constraint equal A5 A6
  constraint equal A4 A5
  constraint concentric A5 A9
  constraint concentric A6 A10
  constraint concentric A7 A11
  constraint equal A10 A11
  constraint equal A9 A10
  constraint equal A8 A9
  constraint coincident P1 P0
  constraint horizontal L30
  constraint perpendicular L30 L31
  constraint parallel L30 L33
  constraint parallel L31 L32
  constraint coincident P4 L27
  constraint coincident P4 L25
  constraint horizontal L28
  constraint perpendicular L26 L28
  constraint parallel L28 L29
  constraint parallel L23 L26
  constraint coincident P4 L24
  constraint coincident P4 L34
  constraint coincident L23.end L24.start
  constraint coincident A13.centre L26.start
  constraint coincident A14.centre L24.end
  constraint coincident A12.centre L23.start
  constraint equal A14 A19
  constraint equal A13 A14
  constraint equal A13 A16
  constraint concentric A13 A15
  constraint concentric A14 A17
  constraint concentric A12 A19
  constraint equal A12 A17
  constraint equal A15 A17
  constraint equal A15 A18
  constraint coincident P4 P3
  constraint coincident L35.end L37.start
  constraint coincident L36.end L37.end
  constraint coincident L36.start L38.start
  constraint coincident L35.start L38.end
  constraint midpoint L37 P4
  measures "d111" distance of L5.end L6.end
  measures "d112" distance of L4.end L5.end
  measures "d113" distance of L10.end L11.end
  measures "d114" distance of L5.end L10.start
  measures "d115" distance of L10.start L10.end
  measures "d116" distance of L5.end L15.end
  measures "d117" distance of L5.end L13.end
  measures "d118" distance of L18.end L19.end
  measures "d119" distance of L17.end L18.end
  measures "d122" diameter of A4
  measures "d136" distance of L27.end L25.end
  measures "d137" distance of L27.end L25.start
  measures "d143" distance of A14.centre A12.centre
  measures "d144" distance of A13.centre A14.centre
  measures "d145" diameter of A16
extrude "Extrude4'" add sketch "Sketch4 (2)" along normal blind 6 contours L3 L5 L6 A9 | L5 L6 A9 | L3 L4 L5 A10 | L6 L7 A8 | L6 L7 A8 | L4 L5 A10 | L4 L7 A11 | L4 L7 A11 bodies 3 in component "Case"
sketch "Sketch5" plane through (66.55, 0, 0) normal (1, 0, 0) x (0, 1, 0) in component "Case"
  line L0 (93.125, -5) -> (-33.075, -5)
  line L1 (-33.075, -5) -> (-33.075, -76)
  line L2 (-33.075, -76) -> (93.125, -76)
  line L3 (93.125, -76) -> (93.125, -5)
  line L4 (74.1111, -71) -> (65.1111, -71)
  line L5 (69.6111, -71) -> (69.6111, -51) construction
  line L6 (76.1111, -55) -> (63.1111, -55)
  line L7 (63.1111, -55) -> (63.1111, -47)
  line L8 (63.1111, -47) -> (76.1111, -47)
  line L9 (76.1111, -47) -> (76.1111, -55)
  line L10 (76.1111, -55) -> (63.1111, -47) construction
  line L11 (63.1111, -55) -> (76.1111, -47) construction
  point P0 (69.6111, -51)
  dimension "d126" = 20
  dimension "d127" = 13
  dimension "d128" = 8
  constraint midpoint L4 L5.start
  constraint perpendicular L4 L5
  constraint horizontal L6
  constraint perpendicular L6 L7
  constraint parallel L6 L8
  constraint parallel L7 L9
  constraint coincident L10 P0
  constraint coincident L11 P0
  constraint coincident P0 L5.end
  measures "d126" distance of L5.start P0
  measures "d127" distance of L7.end L8.end
  measures "d128" distance of L6.end L7.end
extrude "Extrude5" cut sketch "Sketch5" against normal up to surface (5 mm away) contours L6 L7 L8 L9 bodies 3 in component "Case"
sketch "Sketch6" plane through (0, -36.075, 0) normal (0, -1, 0) x (1, 0, 0) in component "Case"
  line L0 (63.55, -5) -> (-25.45, -5)
  line L1 (-25.45, -5) -> (-25.45, -76)
  line L2 (-25.45, -76) -> (63.55, -76)
  line L3 (63.55, -76) -> (63.55, -5)
  line L4 (63.55, -40.5) -> (-25.45, -40.5) construction
  line L5 (-4.75, -39.2) -> (42.85, -39.2)
  line L6 (42.85, -39.2) -> (42.85, -41.8)
  line L7 (42.85, -41.8) -> (-4.75, -41.8)
  line L8 (-4.75, -41.8) -> (-4.75, -39.2)
  line L9 (-4.75, -39.2) -> (42.85, -41.8) construction
  line L10 (42.85, -39.2) -> (-4.75, -41.8) construction
  line L11 (-15.45, -66) -> (53.55, -66) construction
  line L12 (53.55, -66) -> (53.55, -15) construction
  line L13 (53.55, -15) -> (-15.45, -15) construction
  line L14 (-15.45, -15) -> (-15.45, -66) construction
  circle A0 centre (-15.45, -15) radius 2.3
  circle A1 centre (53.55, -15) radius 2.3
  circle A2 centre (53.55, -66) radius 2.3
  circle A3 centre (-15.45, -66) radius 2.3
  point P0 (19.05, -40.5)
  point P1 (19.05, -40.5)
  dimension "d131" = 47.6
  dimension "d132" = 2.6
  dimension "d151" = -10
  dimension "d152" = 4.6
  constraint midpoint L3 L4.start
  constraint midpoint L1 L4.end
  constraint midpoint L4 P1
  constraint horizontal L5
  constraint perpendicular L5 L6
  constraint parallel L5 L7
  constraint parallel L6 L8
  constraint coincident L9 P1
  constraint coincident L10 P1
  constraint coincident P1 P0
  constraint coincident L13.end L14.start
  constraint coincident L12.end L13.start
  constraint coincident L11.end L12.start
  constraint coincident L11.start L14.end
  constraint equal A2 A3
  constraint equal A1 A2
  constraint equal A0 A1
  measures "d131" distance of L6.end L7.end
  measures "d132" distance of L5.end L6.end
  measures "d152" diameter of A0
extrude "Extrude6" cut sketch "Sketch6" against normal up to surface (5 mm away) contours L5 L6 L7 L8 | A0 | A1 | A2 | A3 bodies 3 in component "Case"
extrude "Extrude7" add sketch "Sketch4 (2)" along normal blind 12.5 contours A12 L30 L32 | A12 L30 L32 | A17 L30 L31 | A17 L30 L31 | A18 L32 L33 | A18 L32 L33 | A15 L31 L33 | A15 L31 L33 | A13 | A14 | A16 | A19 bodies 3 in component "Case"
sketch "Sketch7" plane through (0, 0, -58.5) normal (0, 0, 1) x (-1, 0, 0) in component "Case"
  circle A0 centre (13.855, -32.045) radius 3.65
  circle A1 centre (13.855, -6.055) radius 3.65
  circle A2 centre (-51.955, -6.055) radius 3.65
  circle A3 centre (-51.955, -32.045) radius 3.65
  circle A4 centre (13.855, -32.045) radius 1.15
  circle A5 centre (13.855, -6.055) radius 1.15
  circle A6 centre (-51.955, -6.055) radius 1.15
  circle A7 centre (-51.955, -32.045) radius 1.15
  dimension "d148" = 2.3
  constraint concentric A0 A4
  constraint concentric A1 A5
  constraint concentric A2 A6
  constraint concentric A3 A7
  constraint equal A5 A6
  constraint equal A6 A7
  constraint equal A4 A7
  measures "d148" diameter of A4
extrude "Extrude8" cut sketch "Sketch7" against normal blind 4 contours A4 | A5 | A6 | A7 bodies 3 in component "Case"
sketch "Sketch2 (3)" plane through (0, 0, 0) normal (0, 0, 1) x (1, 0, 0) in component "DipPlate"
  line L0 (32.905, -12.995) -> (-32.905, -12.995) construction
  line L1 (-32.905, -12.995) -> (-32.905, 12.995) construction
  line L2 (-32.905, 12.995) -> (32.905, 12.995) construction
  line L3 (32.905, 12.995) -> (32.905, -12.995) construction
  line L4 (32.905, -12.995) -> (-32.905, 12.995) construction
  line L5 (-32.905, -12.995) -> (32.905, 12.995) construction
  circle A0 centre (-32.905, -12.995) radius 1.15
  circle A1 centre (32.905, -12.995) radius 1.15
  circle A2 centre (32.905, 12.995) radius 1.15
  circle A3 centre (-32.905, 12.995) radius 1.15
  line L6 (35, -15) -> (-35, -15)
  line L7 (-35, -15) -> (-35, 15)
  line L8 (-35, 15) -> (35, 15)
  line L9 (35, 15) -> (35, -15)
  line L10 (35, -15) -> (-35, 15) construction
  line L11 (-35, -15) -> (35, 15) construction
  line L12 (21.29, -5.4) -> (-23.71, -5.4)
  line L13 (21.29, -5.4) -> (21.29, 5.4)
  line L14 (21.29, 5.4) -> (-23.71, 5.4)
  line L15 (-23.71, 5.4) -> (-23.71, -5.4)
  line L16 (21.29, 0) -> (-23.71, 0) construction
  line L17 (-23.71, -5.4) -> (21.29, 5.4) construction
  line L18 (21.29, -5.4) -> (-23.71, 5.4) construction
  line L19 (66.55, 93.125) -> (66.55, -33.075) construction
  line L20 (-28.45, -33.075) -> (-28.45, 93.125) construction
  line L21 (21.29, -2.4) -> (18.29, -2.4) construction
  line L22 (18.29, -2.4) -> (18.29, -5.4) construction
  circle A4 centre (32.905, 12.995) radius 3.65
  circle A5 centre (-32.905, 12.995) radius 3.65
  circle A6 centre (-32.905, -12.995) radius 3.65
  circle A7 centre (32.905, -12.995) radius 3.65
  line L23 (-48.71, -23) -> (46.29, -23)
  line L24 (46.29, -23) -> (46.29, 23)
  line L25 (46.29, 23) -> (-48.71, 23)
  line L26 (-48.71, 23) -> (-48.71, -23)
  line L27 (-48.71, -23) -> (46.29, 23) construction
  line L28 (46.29, -23) -> (-48.71, 23) construction
  line L29 (-28.45, 93.125) -> (66.55, 93.125) construction
  line L30 (-29.255, 23) -> (-29.255, -23)
  line L31 (29.255, -23) -> (29.255, 23)
  line L32 (-35, 0) -> (-48.71, 0) construction
  circle A8 centre (-40, 0) radius 3.075
  line L33 (-44, -6.5) -> (-36, -6.5)
  line L34 (-36, -6.5) -> (-36, 6.5)
  line L35 (-36, 6.5) -> (-44, 6.5)
  line L36 (-44, 6.5) -> (-44, -6.5)
  line L37 (-44, -6.5) -> (-36, 6.5) construction
  line L38 (-36, -6.5) -> (-44, 6.5) construction
  point P0 (-1.21, 0)
  point P1 (-1.21, 0)
  point P2 (-40, 0)
  dimension "d159" = 65.81
  dimension "d160" = 25.99
  dimension "d161" = 2.3
  dimension "d162" = 70
  dimension "d163" = 30
  dimension "d167" = 45
  dimension "d168" = 33.79
  dimension "d169" = 10.8
  dimension "d170" = 3
  dimension "d171" = 2.5
  dimension "d173" = 8
  dimension "d175" = 6.15
  dimension "d182" = 8
  dimension "d183" = 13
  dimension "d222" = 1
  constraint horizontal L0
  constraint perpendicular L0 L1
  constraint parallel L0 L2
  constraint parallel L1 L3
  constraint coincident L4 origin
  constraint coincident L5 origin
  constraint coincident L0.end L1.start
  constraint coincident L0.start L3.end
  constraint coincident L2.end L3.start
  constraint coincident L1.end L2.start
  constraint equal A2 A3
  constraint equal A1 A2
  constraint equal A0 A1
  constraint horizontal L6
  constraint perpendicular L6 L7
  constraint parallel L6 L8
  constraint parallel L7 L9
  constraint coincident L10 origin
  constraint coincident L11 origin
  constraint horizontal L12
  constraint perpendicular L12 L13
  constraint perpendicular L13 L14
  constraint coincident L12 L15.end
  constraint perpendicular L12 L15
  constraint coincident L12.end L15.end
  constraint midpoint L13 L16.start
  constraint midpoint L15 L16.end
  constraint coincident origin L16
  constraint midpoint L16 P1
  constraint coincident L13 L21.start
  constraint perpendicular L13 L21
  constraint coincident L12 L22.end
  constraint perpendicular L12 L22
  constraint equal L21 L22
  constraint concentric A2 A4
  constraint concentric A3 A5
  constraint concentric A0 A6
  constraint equal A4 A7
  constraint equal A4 A5
  constraint equal A5 A6
  constraint horizontal L23
  constraint perpendicular L23 L24
  constraint parallel L23 L25
  constraint parallel L24 L26
  constraint coincident L27 P1
  constraint coincident L28 P1
  constraint coincident L20.end L29.start
  constraint coincident L19.start L29.end
  constraint equal L23 L29
  constraint coincident P1 P0
  constraint coincident L25 L30.start
  constraint coincident L23 L30.end
  constraint perpendicular L23 L30
  constraint coincident L23 L31.start
  constraint coincident L25 L31.end
  constraint perpendicular L25 L31
  constraint tangent A5 L30
  constraint tangent A4 L31
  constraint midpoint L7 L32.start
  constraint midpoint L26 L32.end
  constraint horizontal L33
  constraint perpendicular L33 L34
  constraint parallel L33 L35
  constraint parallel L34 L36
  constraint coincident L37 P2
  constraint coincident L38 P2
  constraint coincident P2 A8.centre
  constraint coincident L32 P2
  measures "d159" distance of L1.end L2.end
  measures "d160" distance of L0.end L1.end
  measures "d161" diameter of A0
  measures "d162" distance of L7.end L8.end
  measures "d163" distance of L6.end L7.end
  measures "d167" distance of L12.start L12.end
  measures "d168" distance of L7 P1
  measures "d169" distance of L14.end L12.end
  measures "d170" distance of L21.start L21.end
  measures "d173" distance of L6 L23
  measures "d175" diameter of A8
  measures "d182" distance of L34.end L35.end
  measures "d183" distance of L33.end L34.end
  measures "d222" distance of L7 L34
extrude "Extrude7'" add sketch "Sketch2 (3)" along normal blind 5.6 separate body contours A0 | A1 | A2 | A3 | L6 L9 A7 | L6 L9 A7 | L6 L8 L9 A4 A7 L23 L24 L25 L31 | L6 A7 L31 | L9 A4 A7 L31 | L6 L23 L30 L31 | L6 L8 L30 L31 | L8 L9 A4 | L8 L9 A4 | L6 L7 L8 A5 A6 L23 L25 L26 L30 | L6 A6 L30 | L8 A4 L31 | L6 L7 A6 | L6 L7 A6 | L7 A5 A6 L30 | L8 L25 L30 L31 | L7 L8 A5 | L8 A5 L30 | L7 L8 A5 | L33 L34 L35 L36 makes body 4 in component "DipPlate"
extrude "Extrude8'" cut sketch "Sketch2 (3)" along normal blind 3 contours L6 L8 L30 L31 bodies 4 in component "DipPlate"
extrude "Extrude9" cut sketch "Sketch2 (3)" along normal blind 4 contours A0 | A1 | A2 | A3 bodies 4 in component "DipPlate"
sketch "Sketch7 (2)" plane through (0, 0, 0) normal (0, 0, 1) x (1, 0, 0) in component "DipPlate"
  circle A0 centre (-40, 0) radius 3.075
  line L0 (21.29, 5.4) -> (21.29, -5.4)
  line L1 (21.29, -5.4) -> (-23.71, -5.4)
  line L2 (-23.71, -5.4) -> (-23.71, 5.4)
  line L3 (-23.71, 5.4) -> (21.29, 5.4)
  line L4 (-48.71, 23) -> (-48.71, -23)
  line L5 (-48.71, -23) -> (46.29, -23)
  line L6 (46.29, -23) -> (46.29, 23)
  line L7 (46.29, 23) -> (-48.71, 23)
  line L8 (-43.71, -18) -> (41.29, -18) construction
  line L9 (41.29, -18) -> (41.29, 18) construction
  line L10 (41.29, 18) -> (-43.71, 18) construction
  line L11 (-43.71, 18) -> (-43.71, -18) construction
  circle A1 centre (41.29, 18) radius 2
  circle A2 centre (41.29, -18) radius 2
  circle A3 centre (-43.71, -18) radius 2
  circle A4 centre (-43.71, 18) radius 2
  dimension "d219" = 4
  constraint coincident L9.end L10.start
  constraint coincident L8.end L9.start
  constraint coincident L8.start L11.end
  constraint coincident L10.end L11.start
  constraint equal A3 A4
  constraint equal A2 A3
  constraint equal A1 A2
  measures "d219" diameter of A4
extrude "Extrude10" cut sketch "Sketch7 (2)" along normal up to surface (5.6 mm away) contours A1 | A2 | A3 | A4 bodies 4 in component "DipPlate"
fillet "Fillet3" radius 3 4 edges at (-48.71, -23, 2.8) (46.29, -23, 2.8) (46.29, 23, 2.8) (-48.71, 23, 2.8) on bodies 4 in component "DipPlate"
component "Plate" placed x (1, 0, 0) y (0, 1, 0) z (0, 0, 1) at (0, 0, 0)
component "Case" placed x (1, 0, 0) y (0, 1, 0) z (0, 0, 1) at (0, 0, 0)
component "DipPlate" placed x (-1, 0, 0) y (0, -1, 0) z (0, 0, 1) at (17.84, -59.075, -5.6)
component "Insert" placed x (1, 0, 0) y (0, 1, 0) z (0, 0, 1) at (0, 0, 0) in component "Plate"
equation "WallThickness = 5 mm"
equation "d24 = 80 mm + ( WallThickness * 2 ) + 5 mm"
equation "d25 = WallThickness * 2"
equation "d32 = M3HoleDiameter"
equation "d35 = WallThickness * 2"
equation "d100 = -WallThickness"
equation "M3InsertDiameter = 4.6 mm"
equation "M3InsertLength = 6 mm"
equation "d103 = M3InsertDiameter"
equation "d105 = M3InsertLength"
equation "d109 = WallThickness"
equation "d118 = 68 mm - 2.19 mm"
equation "d119 = 28.18 mm - 2.19 mm"
equation "M1p6InsertDiameter = 2.3 mm"
equation "M1p6InsertLength = 4 mm"
equation "d122 = M1p6InsertDiameter"
equation "d124 = M3InsertLength"
equation "d126 = M1p6InsertLength + 16 mm"
equation "d143 = 68 mm - 2.19 mm"
equation "d144 = 28.18 mm - 2.19 mm"
equation "d145 = M1p6InsertDiameter"
equation "d148 = M1p6InsertDiameter"
equation "d149 = -M1p6InsertLength"
equation "d161 = M1p6InsertDiameter"
equation "d168 = 5.35 mm + 27.94 mm + 0.5 mm"
equation "d173 = 3 mm + WallThickness"
equation "d214 = M1p6InsertLength"
equation "d216 = -WallThickness"
equation "M3HoleDiameter = 4 mm"
equation "d219 = M3HoleDiameter"
